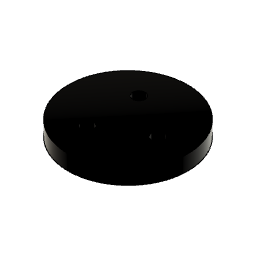
bearing_bottom_cap (Autodesk Fusion 360 design; units mm, degrees)
Autodesk Fusion 360 part; units mm, degrees
sketch "Sketch1" plane through (0, 0, 0) normal (0, 1, 0) x (1, 0, 0)
  circle A0 centre (0, 0) radius 16
  circle A1 centre (8, 0) radius 1.65
  circle A2 centre (-4, 6.9282) radius 1.65
  circle A3 centre (-4, -6.9282) radius 1.65
  dimension "d1" = 32
  dimension "d2" = 3.3
  dimension "d3" = 8
  dimension "d5" = 360
  constraint coincident A0.centre origin
  measures "d1" diameter of A0
  measures "d2" diameter of A1
  measures "d3" distance of A0.centre A1.centre
extrude "Extrude1" add sketch "Sketch1" along normal blind 4
